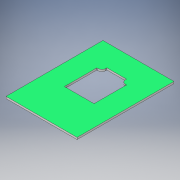
# Autodesk Inventor part: ADIS16448
Saved by Autodesk Inventor 2017 (Build 210142000, 142)
## iProperties
Created: 2016-12-19
Part Number: ADIS16448
Material: Generic
Document SubType Name: Modeling
Designer: Roksbot
Density: 1 g/cm^3
Appearance: Default
Author: Roksbot
Autodesk Inventor part; units mm, degrees
ref_plane "YZ Plane" through (0, 0, 0) normal (1, 0, 0) x (0, 1, 0)
ref_plane "XZ Plane" through (0, 0, 0) normal (0, 1, 0) x (-1, 0, 0)
ref_plane "XY Plane" through (0, 0, 0) normal (0, 0, 1) x (1, 0, 0)
sketch "Sketch1" plane through (0, 0, 0) normal (0, 1, 0) x (-1, 0, 0)
  line L0 (-28.4099, 38.7477) -> (28.4099, 38.7477)
  line L1 (28.4099, 38.7477) -> (28.4099, -38.7477)
  line L2 (28.4099, -38.7477) -> (-28.4099, -38.7477)
  line L3 (-28.4099, -38.7477) -> (-28.4099, 38.7477)
  line L4 (-28.4099, 38.7477) -> (28.4099, -38.7477) construction
  line L5 (28.4099, 38.7477) -> (-28.4099, -38.7477) construction
  point P0 (0, 0)
  dimension "d0" = 56.8198
  dimension "d1" = 77.4954
  constraints: 12 end point, 2 midpoint, 2 parallel, 1 horizontal, 1 perpendicular
  measures "d0" distance of L1.end L2.end
  measures "d1" distance of L0.end L1.end
extrude "Extrusion1" add sketch "Sketch1" along normal blind 1.524
sketch "Sketch2" plane through (0, 1.524, 0) normal (0, 1, 0) x (1, 0, 0)
  line L0 (11.8491, 21.3487) -> (7.8105, 21.3487) construction
  line L1 (-11.8491, 21.3487) -> (-11.8491, 17.3101) construction
  line L2 (-11.8491, -8.6233) -> (11.8491, -8.6233)
  line L3 (11.8491, -8.6233) -> (11.8491, 17.3101)
  line L4 (11.8491, 21.3487) -> (-11.8491, -8.6233) construction
  line L5 (-11.8491, 21.3487) -> (11.8491, -8.6233) construction
  line L6 (28.4099, 38.7477) -> (-28.4099, 38.7477) projected
  line L7 (-15.8877, 25.3873) -> (-7.8105, 25.3873)
  line L8 (-7.8105, 25.3873) -> (-7.8105, 20.4851)
  line L9 (-10.9855, 17.3101) -> (-15.8877, 17.3101)
  line L10 (-15.8877, 17.3101) -> (-15.8877, 25.3873) construction
  line L11 (-15.8877, 25.3873) -> (-7.8105, 17.3101) construction
  line L12 (-7.8105, 25.3873) -> (-15.8877, 17.3101) construction
  line L13 (15.8877, 25.3873) -> (7.8105, 25.3873)
  line L14 (7.8105, 25.3873) -> (7.8105, 21.3487)
  line L15 (10.9855, 17.3101) -> (11.8491, 17.3101)
  line L16 (15.8877, 17.3101) -> (15.8877, 25.3873)
  line L17 (15.8877, 25.3873) -> (7.8105, 17.3101) construction
  line L18 (7.8105, 25.3873) -> (15.8877, 17.3101) construction
  arc A0 (-10.9855, 17.3101) -> (-7.8105, 20.4851) centre (-10.9855, 20.4851) ccw
  arc A1 (7.8105, 20.4851) -> (10.9855, 17.3101) centre (10.9855, 20.4851) ccw
  line L19 (-11.8491, 17.3101) -> (-11.8491, -8.6233)
  line L20 (-7.8105, 21.3487) -> (-11.8491, 21.3487) construction
  line L21 (7.8105, 21.3487) -> (7.8105, 20.4851)
  line L22 (11.8491, 17.3101) -> (15.8877, 17.3101)
  line L23 (7.8105, 21.3487) -> (-7.8105, 21.3487)
  line L24 (11.8491, 17.3101) -> (11.8491, 21.3487) construction
  point P0 (0, 0)
  point P1 (0, 6.3627)
  point P2 (0, 6.3627)
  dimension "d4" = 23.6982
  dimension "d5" = 29.972
  dimension "d6" = 17.399
  dimension "d7" = 4.0386
  dimension "d8" = 4.0386
  dimension "d9" = 3.175
  constraints: 48 end point, 13 parallel, 9 perpendicular, 7 midpoint, 6 point on line, 6 tangent, 5 horizontal, 4 point on circle, 2 centre point, 1 collinear, 1 equal radius, 1 horizontal alignment, 1 vertical alignment
  measures "d4" distance of L0.start L1.start
  measures "d5" distance of L1.start L2.start
  measures "d6" distance between parallel lines of L6 L0
  measures "d7" distance between parallel lines of L1 L8
  measures "d8" distance between parallel lines of L0 L9
  measures "d9" radius of A0
extrude "Extrusion2" cut sketch "Sketch2" against normal through all contours L19 L9 A0 L8 L23 L21 A1 L15 L3 L2
equation "\"d8\" = d7"
body "Solid1"
